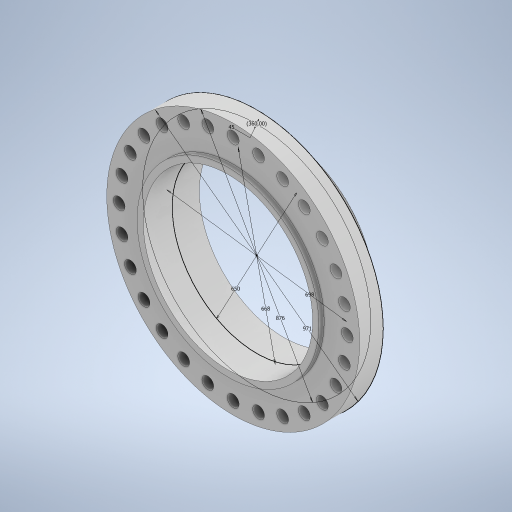
# Autodesk Inventor part: messa in tavola
Saved by Autodesk Inventor 2023 (Build 270158000, 158)
## iProperties
Created: 2023-05-30
Part Number: messa in tavola
Material: Generico
Document SubType Name: Modeling
Designer: Admin
Density: 1 g/cm^3
Appearance: Default
Author: Admin
Autodesk Inventor part; units mm, degrees
ref_plane "YZ Plane" through (0, 0, 0) normal (1, 0, 0) x (0, 1, 0)
ref_plane "XZ Plane" through (0, 0, 0) normal (0, 1, 0) x (-1, 0, 0)
ref_plane "XY Plane" through (0, 0, 0) normal (0, 0, 1) x (1, 0, 0)
sketch "Schizzo1" plane through (0, 0, 0) normal (0, 0, 1) x (1, 0, 0)
  circle A0 centre (0, 0) radius 485.5
  circle A1 centre (0, 0) radius 325
  circle A2 centre (0, 0) radius 334
  circle A3 centre (0, 0) radius 349
  circle A4 centre (0, 0) radius 438 construction
  circle A5 centre (0, 438) radius 22.5
  circle A6 centre (-97.4642, 427.0184) radius 22.5
  circle A7 centre (-190.0411, 394.6244) radius 22.5
  circle A8 centre (-273.0885, 342.4422) radius 22.5
  circle A9 centre (-342.4422, 273.0885) radius 22.5
  circle A10 centre (-394.6244, 190.0411) radius 22.5
  circle A11 centre (-427.0184, 97.4642) radius 22.5
  circle A12 centre (-438, 0) radius 22.5
  circle A13 centre (-427.0184, -97.4642) radius 22.5
  circle A14 centre (-394.6244, -190.0411) radius 22.5
  circle A15 centre (-342.4422, -273.0885) radius 22.5
  circle A16 centre (-273.0885, -342.4422) radius 22.5
  circle A17 centre (-190.0411, -394.6244) radius 22.5
  circle A18 centre (-97.4642, -427.0184) radius 22.5
  circle A19 centre (0, -438) radius 22.5
  circle A20 centre (97.4642, -427.0184) radius 22.5
  circle A21 centre (190.0411, -394.6244) radius 22.5
  circle A22 centre (273.0885, -342.4422) radius 22.5
  circle A23 centre (342.4422, -273.0885) radius 22.5
  circle A24 centre (394.6244, -190.0411) radius 22.5
  circle A25 centre (427.0184, -97.4642) radius 22.5
  circle A26 centre (438, 0) radius 22.5
  circle A27 centre (427.0184, 97.4642) radius 22.5
  circle A28 centre (394.6244, 190.0411) radius 22.5
  circle A29 centre (342.4422, 273.0885) radius 22.5
  circle A30 centre (273.0885, 342.4422) radius 22.5
  circle A31 centre (190.0411, 394.6244) radius 22.5
  circle A32 centre (97.4642, 427.0184) radius 22.5
  dimension "d5" = 876
  dimension "d0" = 971
  dimension "d1" = 650
  dimension "d2" = 668
  dimension "d3" = 698
  dimension "d6" = 45
  dimension "d9" = 360
  constraints: 32 centre point, 5 coincident, 2 vertical alignment, 59 other
  measures "d0" diameter of A0
  measures "d1" diameter of A1
  measures "d2" diameter of A2
  measures "d3" diameter of A3
  measures "d6" diameter of A5
extrude "Estrusione1" add sketch "Schizzo1" along normal blind 90 contours A0
extrude "Estrusione2" add sketch "Schizzo1" along normal blind 110 and the other way blind 105 contours A2 | A3
fillet "Raccordo1" radius 2 1 edges at (-349, 0, -105)
